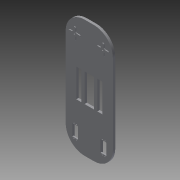
# Autodesk Inventor part: SheepBody
Saved by Autodesk Inventor 2014 SP1 (Build 180222100, 222)
## iProperties
Created: 2013-09-20
Part Number: SheepBody
Material: Generic
Document SubType Name: Modeling
Designer: Medrimonia
Density: 1 g/cm^3
Appearance: Default
ServoTraceSpacing: 0,500 mm
d73: 11,400 mm
d74: 23,500 mm
d77: 4,400 mm
d114: 11,400 mm
d115: 23,500 mm
d116: 3,000 mm
d117: 2,400 mm
d118: 4,400 mm
d121: 2,600 mm
d131: 11,400 mm
d132: 23,500 mm
d133: 4,400 mm
ServoArmWidth: 4,900 mm
ServoArmSpacing: 0,200 mm
ServoArmLength: 10,200 mm
ServoArmThickness: 1,900 mm
ServoArmHoleRequired: 3,000 mm
ServoArmHeadScrewTrace: 5,500 mm
ServoArmHeadScrewThickness: 0,500 mm
MinimalThickness: 2,000 mm
ServoArmInternFillet: 2,000 mm
ServoArmExternFillet: 2,450 mm
ServoCoreToFixation: 2,400 mm
ServoEdgeToFixation: 3,000 mm
ServoCoreWidth: 11,400 mm
ServoSpacing: 0,200 mm
ServoCoreLength: 23,500 mm
ServoFixationLength: 4,400 mm
ServoScrewDiameter: 2,000 mm
ServoScrewDiameterRequired: 2,600 mm
ServoHeadScrewTrace: 4,500 mm
ServoHeadScrewThickness: 2,500 mm
ServoExtendedSpacing: 1,000 mm
ServoAxisToCenter: 6,500 mm
BodyServoThickness: 3,000 mm
d149: 11,400 mm
d150: 23,500 mm
d151: 3,000 mm
d153: 4,400 mm
d154: 0,500 mm
d155: 0,500 mm
d158: 11,400 mm
d159: 23,500 mm
d160: 3,000 mm
d162: 4,400 mm
d183: 11,400 mm
d184: 23,500 mm
d185: 4,400 mm
d186: 0,500 mm
d187: 0,500 mm
d189: 11,400 mm
d190: 23,500 mm
d191: 4,400 mm
d206: 4,900 mm
d207: 4,900 mm
d208: 10,200 mm
d209: 3,000 mm
Author: Medrimonia
Autodesk Inventor part; units mm, degrees
ref_plane "YZ Plane" through (0, 0, 0) normal (1, 0, 0) x (0, 1, 0)
ref_plane "XZ Plane" through (0, 0, 0) normal (0, 1, 0) x (-1, 0, 0)
ref_plane "XY Plane" through (0, 0, 0) normal (0, 0, 1) x (1, 0, 0)
sketch "BodySketch" plane through (0, 0, 0) normal (0, 1, 0) x (-1, 0, 0)
  line L0 (-50, 125) -> (50, 125)
  line L1 (50, 125) -> (50, -125)
  line L2 (50, -125) -> (-50, -125)
  line L3 (-50, -125) -> (-50, 125)
  line L4 (0, 0) -> (109.854, 0) construction
  line L5 (0, 0) -> (0, -80.4744) construction
  dimension "d145" = 100
  dimension "d146" = 250
  constraints: 12 end point, 3 parallel, 2 perpendicular, 1 horizontal, 2 other
  measures "d145" distance between parallel lines of L1 L3
  measures "d146" distance between parallel lines of L2 L0
extrude "Body" add sketch "BodySketch" along normal blind 5
sketch "ServoHoles" plane through (0, 5, 0) normal (0, 1, 0) x (1, 0, 0)
  line L0 (50, -125) -> (50, 125) projected
  line L1 (24.3, 101.75) -> (35.7, 101.75) construction
  line L2 (35.7, 101.75) -> (35.7, 78.25) construction
  line L3 (35.7, 78.25) -> (24.3, 78.25) construction
  line L4 (24.3, 78.25) -> (24.3, 101.75) construction
  line L5 (24.3, 101.75) -> (24.3, 106.15) construction
  line L6 (24.3, 106.15) -> (35.7, 106.15) construction
  line L7 (35.7, 106.15) -> (35.7, 101.75) construction
  line L8 (35.7, 78.25) -> (35.7, 73.85) construction
  line L9 (35.7, 73.85) -> (24.3, 73.85) construction
  line L10 (24.3, 73.85) -> (24.3, 78.25) construction
  circle A0 centre (27.3, 104.15) radius 1.3
  line L11 (23.8, 102.25) -> (36.2, 102.25)
  line L12 (36.2, 102.25) -> (36.2, 77.75)
  line L13 (36.2, 77.75) -> (23.8, 77.75)
  line L14 (23.8, 77.75) -> (23.8, 102.25)
  line L15 (30, 69.4505) -> (30, 18.4289) construction
  line L16 (10.1912, 90) -> (43.5028, 90) construction
  circle A1 centre (32.7, 104.15) radius 1.3
  circle A2 centre (27.3, 75.85) radius 1.3
  circle A3 centre (32.7, 75.85) radius 1.3
  line L17 (0, 0) -> (0, 82.4245) construction
  line L18 (0, 0) -> (107.6133, 0) construction
  line L19 (-24.3, 101.75) -> (-35.7, 101.75) construction
  line L20 (-35.7, 101.75) -> (-35.7, 78.25) construction
  line L21 (-35.7, 78.25) -> (-24.3, 78.25) construction
  line L22 (-24.3, 78.25) -> (-24.3, 101.75) construction
  line L23 (-24.3, 101.75) -> (-24.3, 106.15) construction
  line L24 (-24.3, 106.15) -> (-35.7, 106.15) construction
  line L25 (-35.7, 106.15) -> (-35.7, 101.75) construction
  line L26 (-35.7, 78.25) -> (-35.7, 73.85) construction
  line L27 (-35.7, 73.85) -> (-24.3, 73.85) construction
  line L28 (-24.3, 73.85) -> (-24.3, 78.25) construction
  circle A4 centre (-27.3, 104.15) radius 1.3
  line L29 (-23.8, 102.25) -> (-36.2, 102.25)
  line L30 (-36.2, 102.25) -> (-36.2, 77.75)
  line L31 (-36.2, 77.75) -> (-23.8, 77.75)
  line L32 (-23.8, 77.75) -> (-23.8, 102.25)
  line L33 (-30, 69.4505) -> (-30, 18.4289) construction
  line L34 (-10.1912, 90) -> (-43.5028, 90) construction
  circle A5 centre (-32.7, 104.15) radius 1.3
  circle A6 centre (-27.3, 75.85) radius 1.3
  circle A7 centre (-32.7, 75.85) radius 1.3
  dimension "d149" = 11.4
  dimension "d150" = 23.5
  dimension "d151" = 3
  dimension "d153" = 4.4
  dimension "d154" = 0.5
  dimension "d155" = 0.5
  dimension "d166" = 2.4
  dimension "d167" = 2.6
  dimension "d168" = 30
  dimension "d169" = 90
  constraints: 68 end point, 23 symmetric about line, 8 centre point, 8 parallel, 7 perpendicular, 2 horizontal, 1 collinear, 12 other
  measures "d149" distance between parallel lines of L2 L4
  measures "d150" distance between parallel lines of L3 L1
  measures "d151" distance from line of L5 A0.centre
  measures "d153" distance between parallel lines of L1 L6
  measures "d154" distance between parallel lines of L1 L11
  measures "d155" distance between parallel lines of L2 L12
  measures "d166" distance from line of A0.centre L1
  measures "d167" diameter of A0
  measures "d168" distance from line of L15 L17.start
  measures "d169" distance from line of L16 L17.start
sketch "Sketch15" plane through (0, 5, 0) normal (0, 1, 0) x (1, 0, 0)
  line L0 (18.8, 27.75) -> (18.8, 52.25) projected
  line L1 (18.8, 52.25) -> (31.2, 52.25) projected
  line L2 (31.2, 52.25) -> (31.2, 27.75) projected
  line L3 (31.2, 27.75) -> (18.8, 27.75) projected
  circle A0 centre (-27.7, 25.85) radius 1.3 projected
  circle A1 centre (-22.3, 54.15) radius 1.3 projected
  circle A2 centre (22.3, 25.85) radius 1.3 projected
  circle A3 centre (22.3, 54.15) radius 1.3 projected
  circle A4 centre (27.7, 54.15) radius 1.3 projected
  circle A5 centre (27.7, 25.85) radius 1.3 projected
  circle A6 centre (-27.7, 54.15) radius 1.3 projected
  circle A7 centre (-22.3, 25.85) radius 1.3 projected
  line L4 (-18.8, 27.75) -> (-31.2, 27.75) projected
  line L5 (24.3, 101.75) -> (35.7, 101.75) construction
  line L6 (35.7, 101.75) -> (35.7, 78.25) construction
  line L7 (35.7, 78.25) -> (24.3, 78.25) construction
  line L8 (24.3, 78.25) -> (24.3, 101.75) construction
  line L9 (30, 84.5161) -> (30, -79.0915) construction
  line L10 (24.3, 101.75) -> (24.3, 106.15) construction
  line L11 (24.3, 106.15) -> (35.7, 106.15) construction
  line L12 (35.7, 106.15) -> (35.7, 101.75) construction
  line L13 (35.7, 78.25) -> (35.7, 73.85) construction
  line L14 (35.7, 73.85) -> (24.3, 73.85) construction
  line L15 (24.3, 73.85) -> (24.3, 78.25) construction
  line L16 (-1.6945, 90) -> (27.2352, 90) construction
  line L17 (23.8, 106.65) -> (36.2, 106.65)
  line L18 (36.2, 106.65) -> (36.2, 73.35)
  line L19 (36.2, 73.35) -> (23.8, 73.35)
  line L20 (23.8, 73.35) -> (23.8, 106.65)
  line L21 (30, 0) -> (30, 87.3483) construction
  line L22 (0, 0) -> (75.0033, 0) construction
  line L23 (0, 0) -> (0, 110.6198) construction
  line L24 (-18.8, 27.75) -> (-18.8, 52.25)
  line L25 (-18.8, 52.25) -> (-31.2, 52.25)
  line L26 (-31.2, 52.25) -> (-31.2, 27.75)
  line L27 (-31.2, 27.75) -> (-18.8, 27.75)
  circle A8 centre (-22.3, 25.85) radius 1.3
  circle A9 centre (-22.3, 54.15) radius 1.3
  circle A10 centre (-27.7, 54.15) radius 1.3
  circle A11 centre (-27.7, 25.85) radius 1.3
  line L28 (-24.3, 101.75) -> (-35.7, 101.75) construction
  line L29 (-35.7, 101.75) -> (-35.7, 78.25) construction
  line L30 (-35.7, 78.25) -> (-24.3, 78.25) construction
  line L31 (-24.3, 78.25) -> (-24.3, 101.75) construction
  line L32 (-24.3, 101.75) -> (-24.3, 106.15) construction
  line L33 (-24.3, 106.15) -> (-35.7, 106.15) construction
  line L34 (-35.7, 106.15) -> (-35.7, 101.75) construction
  line L35 (-35.7, 78.25) -> (-35.7, 73.85) construction
  line L36 (-35.7, 73.85) -> (-24.3, 73.85) construction
  line L37 (-24.3, 73.85) -> (-24.3, 78.25) construction
  line L38 (-23.8, 106.65) -> (-36.2, 106.65)
  line L39 (-36.2, 106.65) -> (-36.2, 73.35)
  line L40 (-36.2, 73.35) -> (-23.8, 73.35)
  line L41 (-23.8, 73.35) -> (-23.8, 106.65)
  line L42 (0, 0) -> (-75.0033, 0) construction
  line L43 (-31.2, 27.75) -> (-31.2, 52.25) projected
  line L44 (-31.2, 52.25) -> (-18.8, 52.25) projected
  line L45 (-18.8, 52.25) -> (-18.8, 27.75) projected
  dimension "d183" = 11.4
  dimension "d184" = 23.5
  dimension "d185" = 4.4
  dimension "d186" = 0.5
  dimension "d187" = 0.5
  dimension "d194" = 30
  dimension "d195" = 90
  constraints: 76 end point, 17 symmetric about line, 9 parallel, 7 perpendicular, 4 centre point, 2 collinear, 2 horizontal, 1 coincident, 9 other
  measures "d183" distance between parallel lines of L6 L8
  measures "d184" distance between parallel lines of L7 L5
  measures "d185" distance between parallel lines of L5 L11
  measures "d186" distance between parallel lines of L6 L18
  measures "d187" distance between parallel lines of L11 L17
  measures "d194" distance between parallel lines of L9 L23
  measures "d195" distance between parallel lines of L22 L16
ref_plane "Work Plane9" through (0, 3, 0) normal (0, -1, 0) x (1, 0, 0)
ref_plane "Work Plane10" through (0, 5, 0) normal (0, 1, 0) x (1, 0, 0)
extrude "Extrusion15" cut sketch "ServoHoles" against normal through all
extrude "Extrusion16" cut sketch "Sketch15" along normal up to surface (2 mm away) from surface at -2 contours L17 L18 L19 L20 | L41 L40 L39 L38
sketch "Sketch16" plane through (0, 0, 0) normal (0, -1, 0) x (1, 0, 0)
  line L0 (42.65, 87.55) -> (42.65, 92.45)
  line L1 (17.35, 92.45) -> (17.35, 87.55)
  line L2 (17.35, 87.55) -> (42.65, 92.45) construction
  line L3 (42.65, 87.55) -> (17.35, 92.45) construction
  line L4 (27.55, 77.35) -> (32.45, 77.35)
  line L5 (32.45, 102.65) -> (27.55, 102.65)
  line L6 (27.55, 77.35) -> (32.45, 102.65) construction
  line L7 (32.45, 77.35) -> (27.55, 102.65) construction
  line L8 (42.65, 92.45) -> (32.45, 92.45)
  line L9 (27.55, 92.45) -> (17.35, 92.45)
  line L10 (32.45, 77.35) -> (32.45, 87.55)
  line L11 (32.45, 92.45) -> (32.45, 102.65)
  line L12 (17.35, 87.55) -> (27.55, 87.55)
  line L13 (32.45, 87.55) -> (42.65, 87.55)
  line L14 (27.55, 102.65) -> (27.55, 92.45)
  line L15 (27.55, 87.55) -> (27.55, 77.35)
  circle A0 centre (30, 90) radius 1.5
  line L16 (0, 0) -> (82.9119, 0) construction
  line L17 (0, 0) -> (0, 87.5833) construction
  line L18 (-42.65, 87.55) -> (-42.65, 92.45)
  line L19 (-17.35, 92.45) -> (-17.35, 87.55)
  line L20 (-17.35, 87.55) -> (-42.65, 92.45) construction
  line L21 (-42.65, 87.55) -> (-17.35, 92.45) construction
  line L22 (-27.55, 77.35) -> (-32.45, 77.35)
  line L23 (-32.45, 102.65) -> (-27.55, 102.65)
  line L24 (-27.55, 77.35) -> (-32.45, 102.65) construction
  line L25 (-32.45, 77.35) -> (-27.55, 102.65) construction
  line L26 (-42.65, 92.45) -> (-32.45, 92.45)
  line L27 (-27.55, 92.45) -> (-17.35, 92.45)
  line L28 (-32.45, 77.35) -> (-32.45, 87.55)
  line L29 (-32.45, 92.45) -> (-32.45, 102.65)
  line L30 (-17.35, 87.55) -> (-27.55, 87.55)
  line L31 (-32.45, 87.55) -> (-42.65, 87.55)
  line L32 (-27.55, 102.65) -> (-27.55, 92.45)
  line L33 (-27.55, 87.55) -> (-27.55, 77.35)
  circle A1 centre (-30, 90) radius 1.5
  dimension "d206" = 4.9
  dimension "d207" = 4.9
  dimension "d208" = 10.2
  dimension "d209" = 3
  dimension "d213" = 30
  dimension "d214" = 90
  constraints: 68 end point, 14 symmetric about line, 12 midpoint, 10 parallel, 6 perpendicular, 5 equal length, 3 horizontal, 2 centre point, 1 other
  measures "d206" distance of L5.start L5.end
  measures "d207" distance of L0.start L0.end
  measures "d208" distance of L0.end L8.end
  measures "d209" diameter of A0
  measures "d213" distance from line of L17 point (30, 90)
  measures "d214" distance from line of L16 A0.centre
extrude "Extrusion17" add sketch "Sketch16" along normal blind 1.9
hole "Hole1" at (-30, 0, 90) direction (0, 1, 0) diameter 3 end through all
hole "Hole2" at (30, 0, 90) direction (0, 1, 0) diameter 3 end through all
fillet "Fillet8" radius 2.45 16 edges at (27.55, -0.95, 102.65) (32.45, -0.95, 102.65) (-17.35, -0.95, 92.45) (-27.55, -0.95, 102.65) (-32.45, -0.95, 102.65) (42.65, -0.95, 92.45) (17.35, -0.95, 92.45) (-42.65, -0.95, 92.45) (-42.65, -0.95, 87.55) (-32.45, -0.95, 77.35) (-27.55, -0.95, 77.35) (-17.35, -0.95, 87.55) (17.35, -0.95, 87.55) (27.55, -0.95, 77.35) (32.45, -0.95, 77.35) (42.65, -0.95, 87.55)
chamfer "Chamfer5" distance 2 angle 45 1 edges at (27.55, -0.95, 87.55)
chamfer "Chamfer6" distance 2 angle 45 3 edges at (27.55, -0.95, 92.45) (32.45, -0.95, 92.45) (32.45, -0.95, 87.55)
chamfer "Chamfer7" distance 2 angle 45 4 edges at (-32.45, -0.95, 92.45) (-32.45, -0.95, 87.55) (-27.55, -0.95, 87.55) (-27.55, -0.95, 92.45)
fillet "Fillet9" radius 40 4 edges at (-50, 2.5, -125) (50, 2.5, -125) (-50, 2.5, 125) (50, 2.5, 125)
sketch "Sketch17" plane through (0, 0, 0) normal (0, -1, 0) x (1, 0, 0)
  line L0 (-27.5, 30) -> (27.5, 30)
  line L1 (27.5, 30) -> (27.5, -30)
  line L2 (27.5, -30) -> (-27.5, -30)
  line L3 (-27.5, -30) -> (-27.5, 30)
  line L4 (0, 0) -> (106.1682, 0) construction
  line L5 (0, 0) -> (0, 67.4734) construction
  line L6 (10, 30) -> (17, 30) construction
  line L7 (17, -30) -> (10, -30) construction
  line L8 (10, 30) -> (17, 30)
  line L9 (17, 30) -> (17, -30)
  line L10 (17, -30) -> (10, -30)
  line L11 (10, -30) -> (10, 30)
  line L12 (-17, 30) -> (-10, 30)
  line L13 (-10, 30) -> (-10, -30)
  line L14 (-10, -30) -> (-17, -30)
  line L15 (-17, -30) -> (-17, 30)
  dimension "d246" = 55
  dimension "d247" = 60
  dimension "d250" = 7
  dimension "d251" = 10
  dimension "d252" = 7
  dimension "d253" = 10
  constraints: 32 end point, 7 parallel, 6 point on line, 5 perpendicular, 4 horizontal, 2 other
  measures "d246" distance between parallel lines of L1 L3
  measures "d247" distance between parallel lines of L0 L2
  measures "d250" distance between parallel lines of L9 L11
  measures "d251" distance between parallel lines of L5 L11
  measures "d252" distance between parallel lines of L13 L15
  measures "d253" distance between parallel lines of L5 L13
extrude "Extrusion18" cut sketch "Sketch17" against normal through all contours L0 L15 L2 L3 | L0 L11 L2 L13 | L0 L1 L2 L9
equation "\"d145\" = BodyWidth"
equation "\"d146\" = BodyLength"
equation "\"d147\" = BodyThickness"
equation "\"d149\" = ServoCoreWidth"
equation "\"d150\" = ServoCoreLength"
equation "\"d151\" = ServoEdgeToFixation"
equation "\"d153\" = d162"
equation "\"d154\" = ServoTraceSpacing"
equation "\"d155\" = ServoTraceSpacing"
equation "\"d166\" = ServoCoreToFixation"
equation "\"d168\" = BodyServoWidthShift"
equation "\"d169\" = BodyServoLengthShift"
equation "\"ServoTraceSpacing\" = 0.5"
equation "\"BodyServoThickness\" = 3"
equation "\"BodyLength\" = 250"
equation "\"BodyWidth\" = 100"
equation "\"BodyThickness\" = 5"
equation "\"BodyServoWidthShift\" = 30"
equation "\"BodyServoLengthShift\" = 90"
equation "\"BoardHoleWidth\" = 55"
equation "\"BoardHoleSupportWidth\" = 7"
equation "\"ServoCoreWidth\" = 11.4"
equation "\"ServoCoreLength\" = 23.5"
equation "\"ServoEdgeToFixation\" = 3"
equation "\"d162\" = 4.4"
equation "\"ServoCoreToFixation\" = 2.4"
body "Solid2"
